Autodesk Fusion 360 part; units mm, degrees
(part 2 of 2)
sketch "Sketch38" plane through (0, 0, -13) normal (0, 0, -1) x (1, 0, 0)
  line L0 (11.5986, 30.4363) -> (28.0634, 30.4363)
  line L1 (28.0634, 30.4363) -> (20.0901, 16.1809)
  line L2 (20.0901, 16.1809) -> (11.5986, 30.4363)
  arc A0 (36.6796, 36.8191) -> (36.3132, 34) centre (30.5628, 36.1807) ccw
  line L3 (36.6796, 36.8191) -> (40.3994, 36.8191)
  line L4 (40.3994, 36.8191) -> (40.3994, 34)
  line L5 (40.3994, 34) -> (36.3132, 34)
  arc A1 (13.965, 45.3815) -> (14.188, 48) centre (20.0628, 46.1807) ccw
  line L6 (13.965, 45.3815) -> (10, 45.3815)
  line L7 (10, 45.3815) -> (10, 48)
  line L8 (10, 48) -> (14.188, 48)
  line L9 (-13.9372, 19.6807) -> (-27.9372, 19.6807)
  line L10 (-27.9372, 19.6807) -> (-27.9372, 28.6807)
  line L11 (-27.9372, 28.6807) -> (-36.9372, 28.6807)
  line L12 (-36.9372, 28.6807) -> (-36.9372, 42.6807)
  line L13 (-36.9372, 42.6807) -> (-27.9372, 42.6807)
  line L14 (-27.9372, 42.6807) -> (-27.9372, 51.6807)
  line L15 (-27.9372, 51.6807) -> (-13.9372, 51.6807)
  line L16 (-13.9372, 51.6807) -> (-13.9372, 42.6807)
  line L17 (-13.9372, 42.6807) -> (-4.9372, 42.6807)
  line L18 (-4.9372, 42.6807) -> (-4.9372, 28.6807)
  line L19 (-4.9372, 28.6807) -> (-13.9372, 28.6807)
  line L20 (-13.9372, 28.6807) -> (-13.9372, 19.6807)
  line L21 (49.5628, -49.8193) -> (49.5628, 21.1807)
  line L22 (49.5628, 21.1807) -> (52.5628, 21.1807)
  line L23 (52.5628, 21.1807) -> (52.5628, 23.1807)
  line L24 (52.5628, 23.1807) -> (53.5628, 23.1807)
  line L25 (53.5628, 23.1807) -> (53.5628, 34.1807)
  line L26 (53.5628, 34.1807) -> (52.5628, 34.1807)
  line L27 (52.5628, 34.1807) -> (52.5628, 36.1807)
  line L28 (52.5628, 36.1807) -> (49.5628, 36.1807)
  line L29 (49.5628, 36.1807) -> (49.5628, 63.1807)
  line L30 (49.5628, 63.1807) -> (-50.4372, 63.1807)
  line L31 (-50.4372, 63.1807) -> (-50.4372, 28.6807)
  line L32 (-50.4372, 28.6807) -> (-53.4372, 28.6807)
  line L33 (-53.4372, 28.6807) -> (-53.4372, 6.6807)
  line L34 (-53.4372, 6.6807) -> (-50.4372, 6.6807)
  line L35 (-50.4372, 6.6807) -> (-50.4372, -49.8193)
  line L36 (-50.4372, -49.8193) -> (49.5628, -49.8193)
  line L37 (-43.9372, 9.6807) -> (45.0628, 9.6807)
  line L38 (45.0628, 9.6807) -> (45.0628, -48.3193)
  line L39 (45.0628, -48.3193) -> (-43.9372, -48.3193)
  line L40 (-43.9372, -48.3193) -> (-43.9372, 9.6807)
  circle A2 centre (38.0489, 54.1652) radius 6
  circle A3 centre (-39.0183, 55.1346) radius 6
  dimension "d302" = 12
  dimension "d303" = 12
  measures "d302" diameter of A2
  measures "d303" diameter of A3
extrude "Extrude46" add sketch "Sketch38" along normal up to surface (4 mm away) contours A2 | A3 bodies 8
sketch "Sketch39" plane through (0, 0, 2) normal (0, 0, 1) x (-1, 0, 0)
  circle A0 centre (-14.2626, -8.1194) radius 2.45
  circle A1 centre (-14.2626, -8.1194) radius 5.5
  line L0 (-5, 0) -> (-25.2466, 0)
  line L1 (-25.2466, 0) -> (-25.2466, -5.7054)
  line L2 (-25.2466, -5.7054) -> (-5, -5.7054)
  line L3 (-5, -5.7054) -> (-5, 0)
  line L4 (45.9289, 51.2064) -> (28.0993, 51.2064)
  line L5 (28.0993, 51.2064) -> (28.0993, 45.9289)
  line L6 (28.0993, 45.9289) -> (45.9289, 45.9289)
  line L7 (45.9289, 45.9289) -> (45.9289, 51.2064)
  constraint horizontal L0
  constraint vertical L1
  constraint horizontal L2
  constraint vertical L3
  constraint horizontal L4
  constraint vertical L5
  constraint horizontal L6
  constraint vertical L7
extrude "Extrude47" cut sketch "Sketch39" against normal blind 10 contours A0 A1 L2 | A1 L0 L1 L2 L3 | L4 L5 L6 L7 picked at (-13.5808, -3.6987) bodies 7
sketch "Sketch40" plane through (0, 0, 2) normal (0, 0, 1) x (-1, 0, 0)
  line L0 (-14.6811, -5.7054) -> (-19.2045, -5.7054)
  arc A0 (-19.2045, -5.7054) -> (-9.3206, -5.7054) centre (-14.2626, -8.1194) ccw
  line L1 (-9.3206, -5.7054) -> (-13.8441, -5.7054)
  arc A1 (-14.6811, -5.7054) -> (-13.8441, -5.7054) centre (-14.2626, -8.1194) ccw
  line L2 (-33.4231, 51.5144) -> (-47.6815, 51.5144)
  line L3 (-47.6815, 51.5144) -> (-47.6815, 46.7616)
  line L4 (-47.6815, 46.7616) -> (-33.4231, 46.7616)
  line L5 (-33.4231, 46.7616) -> (-33.4231, 51.5144)
  constraint horizontal L2
  constraint vertical L3
  constraint horizontal L4
  constraint vertical L5
extrude "Extrude48" cut sketch "Sketch40" against normal blind 10 contours L2 L3 L4 L5 bodies 7
extrude "Extrude49" cut 1 faces at (-53.1039, 30.1193, -4.5) along direction (0, 0, -1) blind 6.5 on bodies 7 bodies 7
extrude "Extrude50" add 1 faces at (-53.1039, 30.1193, -11) along direction (0, 0, 1) blind 3.5 from surface at 9.5 on bodies 7 bodies 7
extrude "Extrude51" cut 1 faces at (-53.1039, 12.1193, -4.6667) along direction (0, -1, 0) blind 9 on bodies 7 bodies 7
extrude "Extrude52" add 1 faces at (-53.1039, 39.1193, -4.6667) along direction (0, -1, 0) blind 9 on bodies 7 bodies 7
extrude "Extrude53" add 1 faces at (-53.1039, 3.1193, -4.6667) along direction (0, 1, 0) blind 1 on bodies 7 bodies 7
extrude "Extrude54" cut 1 faces at (-53.1039, 30.1193, -4.6667) along direction (0, 1, 0) blind 1 on bodies 7 bodies 7
hidden bodies 1 2 3 5 4 6 8
named bodies: "Body 1", "bottom DO NOT CHOOSE", "done button", "triangle button", "d-pad button", "back button", "Bottom Part (correct)", "Top Part (correct)"
